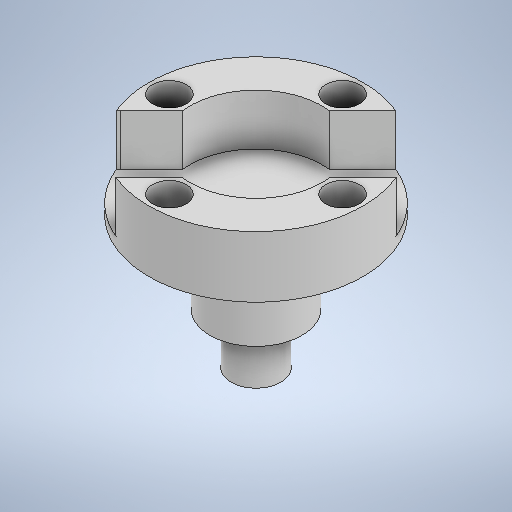
# Autodesk Inventor part: spinner
Saved by Autodesk Inventor 2025.1 (Build 291241000, 241)
## iProperties
Created: 2024-09-30
Part Number: spinner
Material: Generic
Document SubType Name: Modeling
Designer: m_kni
Density: 1 g/cm^3
Appearance: Default
Author: m_kni
Autodesk Inventor part; units mm, degrees
ref_plane "YZ Plane" through (0, 0, 0) normal (1, 0, 0) x (0, 1, 0)
ref_plane "XZ Plane" through (0, 0, 0) normal (0, 1, 0) x (-1, 0, 0)
ref_plane "XY Plane" through (0, 0, 0) normal (0, 0, 1) x (1, 0, 0)
sketch "Sketch1" plane through (0, 0, 0) normal (0, 1, 0) x (-1, 0, 0)
  line L0 (-12.7, 12.7) -> (12.7, 12.7)
  line L1 (12.7, 12.7) -> (12.7, -12.7)
  line L2 (12.7, -12.7) -> (-12.7, -12.7)
  line L3 (-12.7, -12.7) -> (-12.7, 12.7)
  line L4 (-12.7, 12.7) -> (12.7, -12.7) construction
  line L5 (12.7, 12.7) -> (-12.7, -12.7) construction
  line L6 (-11.4786, 11.4786) -> (11.4786, 11.4786)
  line L7 (11.4786, 11.4786) -> (11.4786, -11.4786)
  line L8 (11.4786, -11.4786) -> (-11.4786, -11.4786)
  line L9 (-11.4786, -11.4786) -> (-11.4786, 11.4786)
  line L10 (-11.4786, 11.4786) -> (11.4786, -11.4786) construction
  line L11 (11.4786, 11.4786) -> (-11.4786, -11.4786) construction
  line L12 (-25.4, -25.4) -> (25.4, -25.4)
  line L13 (25.4, -25.4) -> (25.4, 25.4)
  line L14 (25.4, 25.4) -> (-25.4, 25.4)
  line L15 (-25.4, 25.4) -> (-25.4, -25.4)
  line L16 (-25.4, -25.4) -> (25.4, 25.4) construction
  line L17 (25.4, -25.4) -> (-25.4, 25.4) construction
  circle A0 centre (0, 0) radius 5.5
  circle A1 centre (11.4786, 11.4786) radius 5.5
  circle A2 centre (11.4786, -11.4786) radius 5.5
  circle A3 centre (-11.4786, 11.4786) radius 5.5
  circle A4 centre (-11.4786, -11.4786) radius 5.5
  circle A5 centre (-25.4, 25.4) radius 5.5
  circle A6 centre (25.4, 25.4) radius 5.5
  circle A7 centre (25.4, -25.4) radius 5.5
  circle A8 centre (-25.4, -25.4) radius 5.5
  line L18 (7.5895, 15.3677) -> (21.5109, 29.2891)
  line L19 (29.2891, 21.5109) -> (15.3677, 7.5895)
  line L20 (15.3677, -7.5895) -> (29.2891, -21.5109)
  line L21 (-7.5895, -15.3677) -> (-21.5109, -29.2891)
  line L22 (-29.2891, 21.5109) -> (-15.3677, 7.5895)
  line L23 (7.5895, -15.3677) -> (21.5109, -29.2891)
  line L24 (-14.6585, -6.991) -> (-28.5798, -20.9124)
  line L25 (-8.9306, 16.3528) -> (-21.4569, 29.2343)
  line L26 (-35, -35) -> (35, -35)
  line L27 (35, -35) -> (35, 35)
  line L28 (35, 35) -> (-35, 35)
  line L29 (-35, 35) -> (-35, -35)
  line L30 (-35, -35) -> (35, 35) construction
  line L31 (35, -35) -> (-35, 35) construction
  circle A9 centre (11.4786, 11.4786) radius 2.5
  circle A10 centre (25.4, 25.4) radius 2.5
  line L32 (27.1678, 23.6322) -> (13.2464, 9.7109)
  line L33 (23.7072, 27.2397) -> (9.7111, 13.2466)
  line L34 (0, 0) -> (0, 35)
  line L35 (35, 0) -> (0, 0)
  line L36 (-27.1678, 23.6322) -> (-13.2464, 9.7109)
  circle A11 centre (-25.4, 25.4) radius 2.5
  line L37 (-23.7072, 27.2397) -> (-9.7111, 13.2466)
  circle A12 centre (-11.4786, 11.4786) radius 2.5
  circle A13 centre (25.4, -25.4) radius 2.5
  line L38 (23.7072, -27.2397) -> (9.7111, -13.2466)
  line L39 (27.1678, -23.6322) -> (13.2464, -9.7109)
  circle A14 centre (11.4786, -11.4786) radius 2.5
  circle A15 centre (-11.4786, -11.4786) radius 2.5
  line L40 (-23.7072, -27.2397) -> (-9.7111, -13.2466)
  line L41 (-27.1678, -23.6322) -> (-13.2464, -9.7109)
  line L42 (25.4, 25.4) -> (-25.4, -25.4) construction
  circle A16 centre (-25.4, -25.4) radius 2.5
  circle A17 centre (0, 0) radius 10.5
  circle A18 centre (0, 0) radius 6.5
  dimension "d0" = 25.4
  dimension "d1" = 25.4
  dimension "d2" = 50.8
  dimension "d3" = 50.8
  dimension "d4" = 11
  dimension "d5" = 11
  dimension "d6" = 11
  dimension "d7" = 11
  dimension "d8" = 11
  dimension "d9" = 11
  dimension "d10" = 11
  dimension "d11" = 11
  dimension "d12" = 11
  dimension "d13" = 70
  dimension "d14" = 5
  dimension "d15" = 5
  dimension "d16" = 21
  dimension "d17" = 13
  constraints: 86 end point, 32 point on circle, 19 centre point, 18 symmetric about line, 14 coincident, 13 tangent, 10 midpoint, 8 parallel, 5 horizontal, 5 perpendicular, 3 point on line, 6 other
  measures "d0" distance of L1.end L2.end
  measures "d1" distance of L0.end L1.end
  measures "d2" distance of L14.end L13.end
  measures "d3" distance of L13.end L12.end
  measures "d4" diameter of A0
  measures "d5" diameter of A1
  measures "d6" diameter of A2
  measures "d7" diameter of A3
  measures "d8" diameter of A4
  measures "d9" diameter of A5
  measures "d10" diameter of A6
  measures "d11" diameter of A7
  measures "d12" diameter of A8
  measures "d13" distance of L28.end L27.end
  measures "d14" diameter of A9
  measures "d15" diameter of A10
  measures "d16" diameter of A17
  measures "d17" diameter of A18
extrude "Extrusion1" add sketch "Sketch1" along normal blind 8 contours A18 L35 A0 L34 | L34 A0 L35 A18 | L34 L35 A0 | A0 L35 L34
sketch "Sketch2" plane through (0, 8, 0) normal (0, 1, 0) x (1, 0, 0)
  line L0 (-12.7, 12.7) -> (12.7, 12.7)
  line L1 (12.7, 12.7) -> (12.7, -12.7)
  line L2 (12.7, -12.7) -> (-12.7, -12.7)
  line L3 (-12.7, -12.7) -> (-12.7, 12.7)
  line L4 (-12.7, 12.7) -> (12.7, -12.7) construction
  line L5 (12.7, 12.7) -> (-12.7, -12.7) construction
  line L6 (-11.4786, 11.4786) -> (11.4786, 11.4786)
  line L7 (11.4786, 11.4786) -> (11.4786, -11.4786)
  line L8 (11.4786, -11.4786) -> (-11.4786, -11.4786)
  line L9 (-11.4786, -11.4786) -> (-11.4786, 11.4786)
  line L10 (-11.4786, 11.4786) -> (11.4786, -11.4786) construction
  line L11 (11.4786, 11.4786) -> (-11.4786, -11.4786) construction
  line L12 (-25.4, -25.4) -> (25.4, -25.4)
  line L13 (25.4, -25.4) -> (25.4, 25.4)
  line L14 (25.4, 25.4) -> (-25.4, 25.4)
  line L15 (-25.4, 25.4) -> (-25.4, -25.4)
  line L16 (-25.4, -25.4) -> (25.4, 25.4) construction
  line L17 (25.4, -25.4) -> (-25.4, 25.4) construction
  circle A0 centre (0, 0) radius 5.5
  circle A1 centre (11.4786, 11.4786) radius 5.5
  circle A2 centre (11.4786, -11.4786) radius 5.5
  circle A3 centre (-11.4786, 11.4786) radius 5.5
  circle A4 centre (-11.4786, -11.4786) radius 5.5
  circle A5 centre (-25.4, 25.4) radius 5.5
  circle A6 centre (25.4, 25.4) radius 5.5
  circle A7 centre (25.4, -25.4) radius 5.5
  circle A8 centre (-25.4, -25.4) radius 5.5
  line L18 (7.5895, 15.3677) -> (21.5109, 29.2891)
  line L19 (29.2891, 21.5109) -> (15.3677, 7.5895)
  line L20 (15.3677, -7.5895) -> (29.2891, -21.5109)
  line L21 (-7.5895, -15.3677) -> (-21.5109, -29.2891)
  line L22 (-29.2891, 21.5109) -> (-15.3677, 7.5895)
  line L23 (7.5895, -15.3677) -> (21.5109, -29.2891)
  line L24 (-16.1952, -8.6495) -> (-30.1166, -22.5709)
  line L25 (-9.6329, 16.6597) -> (-21.393, 29.1675)
  line L26 (-35, -35) -> (35, -35)
  line L27 (35, -35) -> (35, 35)
  line L28 (35, 35) -> (-35, 35)
  line L29 (-35, 35) -> (-35, -35)
  line L30 (-35, -35) -> (35, 35) construction
  line L31 (35, -35) -> (-35, 35) construction
  circle A9 centre (11.4786, 11.4786) radius 2.5
  circle A10 centre (25.4, 25.4) radius 2.5
  line L32 (27.1678, 23.6322) -> (13.2464, 9.7109)
  line L33 (23.5125, 27.0393) -> (9.7114, 13.247)
  line L34 (0, 0) -> (0, 35)
  line L35 (35, 0) -> (0, 0)
  line L36 (-27.1678, 23.6322) -> (-13.2464, 9.7109)
  circle A11 centre (-25.4, 25.4) radius 2.5
  line L37 (-23.5125, 27.0393) -> (-9.7114, 13.247)
  circle A12 centre (-11.4786, 11.4786) radius 2.5
  circle A13 centre (25.4, -25.4) radius 2.5
  line L38 (23.5125, -27.0393) -> (9.7114, -13.247)
  line L39 (27.1678, -23.6322) -> (13.2464, -9.7109)
  circle A14 centre (11.4786, -11.4786) radius 2.5
  circle A15 centre (-11.4786, -11.4786) radius 2.5
  line L40 (-23.5125, -27.0393) -> (-9.7114, -13.247)
  line L41 (-27.1678, -23.6322) -> (-13.2464, -9.7109)
  line L42 (25.4, 25.4) -> (-25.4, -25.4) construction
  circle A16 centre (-25.4, -25.4) radius 2.5
  circle A17 centre (0, 0) radius 10.5
  dimension "d20" = 25.4
  dimension "d21" = 25.4
  dimension "d22" = 50.8
  dimension "d23" = 50.8
  dimension "d24" = 11
  dimension "d25" = 11
  dimension "d26" = 11
  dimension "d27" = 11
  dimension "d28" = 11
  dimension "d29" = 11
  dimension "d30" = 11
  dimension "d31" = 11
  dimension "d32" = 11
  dimension "d33" = 70
  dimension "d34" = 5
  dimension "d35" = 5
  dimension "d36" = 21
  constraints: 86 end point, 32 point on circle, 18 centre point, 18 symmetric about line, 13 coincident, 13 tangent, 10 midpoint, 8 parallel, 5 horizontal, 5 perpendicular, 3 point on line, 6 other
  measures "d20" distance of L1.end L2.end
  measures "d21" distance of L0.end L1.end
  measures "d22" distance of L14.end L13.end
  measures "d23" distance of L13.end L12.end
  measures "d24" diameter of A0
  measures "d25" diameter of A1
  measures "d26" diameter of A2
  measures "d27" diameter of A3
  measures "d28" diameter of A4
  measures "d29" diameter of A5
  measures "d30" diameter of A6
  measures "d31" diameter of A7
  measures "d32" diameter of A8
  measures "d33" distance of L28.end L27.end
  measures "d34" diameter of A9
  measures "d35" diameter of A10
  measures "d36" diameter of A17
extrude "Extrusion2" add sketch "Sketch2" along normal blind 6 contours A17 L35 A0 L34 | L34 A0 L35 A17 | L34 L35 A0 | A0 L35 L34
sketch "Sketch3" plane through (0, 8, 0) normal (0, -1, 0) x (1, 0, 0)
  circle A0 centre (0, -8.5) radius 1.65
  circle A1 centre (8.5, 0) radius 1.65
  circle A2 centre (-8.5, 0) radius 1.65
  circle A3 centre (0, 8.5) radius 1.65
  point P0 (0, 0)
  dimension "d39" = 8.5
  dimension "d40" = 8.5
  dimension "d41" = 8.5
  dimension "d42" = 8.5
  dimension "d43" = 3.3
  dimension "d44" = 3.3
  dimension "d45" = 3.3
  dimension "d46" = 3.3
  constraints: 4 centre point, 4 coincident
  measures "d39" distance of point (0, -8.5) point (0, 0)
  measures "d40" distance of point (-8.5, 0) point (0, 0)
  measures "d41" distance of point (0, 8.5) point (0, 0)
  measures "d42" distance of point (8.5, 0) point (0, 0)
  measures "d43" diameter of A0
  measures "d44" diameter of A1
  measures "d45" diameter of A2
  measures "d46" diameter of A3
extrude "Extrusion3" cut sketch "Sketch3" against normal blind 6
sketch "Sketch4" plane through (0, 0, 0) normal (0, -1, 0) x (1, 0, 0)
  circle A0 centre (0, 0) radius 2.45
  dimension "d49" = 4.9
  constraints: 1 centre point, 1 coincident
  measures "d49" diameter of A0
extrude "Extrusion4" add sketch "Sketch4" along normal blind 5
sketch "Sketch5" plane through (0, 0, 0) normal (0, -1, 0) x (1, 0, 0)
  circle A0 centre (0, 0) radius 4.5
  circle A1 centre (0, 0) radius 6.5
  dimension "d52" = 9
  constraints: 2 centre point, 2 coincident
  measures "d52" diameter of A0
extrude "Extrusion5" cut sketch "Sketch5" against normal blind 12
sketch "Sketch8" plane through (0, 14, 0) normal (0, 1, 0) x (1, 0, 0)
  circle A0 centre (0, 0) radius 1.5
  circle A1 centre (0, 0) radius 5.6
  line L0 (-8.3358, -3.9626) -> (-17.8155, -2.4306)
  arc A2 (-17.8155, 2.5054) -> (-17.8155, -2.4306) centre (-17.4166, 0.0374) ccw
  line L1 (-8.3358, 4.0374) -> (-17.8155, 2.5054)
  line L2 (8.5026, 4.0374) -> (17.9822, 2.5054)
  arc A3 (17.9822, -2.4306) -> (17.9822, 2.5054) centre (17.5834, 0.0374) ccw
  line L3 (8.5026, -3.9626) -> (17.9822, -2.4306)
  line L4 (-8.3358, 4.0374) -> (-17.8155, 2.5054)
  line L5 (-17.8155, -2.4306) -> (-8.3358, -3.9626)
  line L6 (17.9822, 2.5054) -> (8.5026, 4.0374)
  line L7 (8.5026, -3.9626) -> (17.9822, -2.4306)
  circle A4 centre (17.5834, 0.0374) radius 2.5
  circle A5 centre (-17.4166, 0.0374) radius 2.5
  circle A6 centre (0, 0) radius 10.5
  line L8 (-3.0923, -8.6963) -> (-4.0736, -9.6776)
  line L9 (-8.7492, -3.0394) -> (-9.7087, -3.999)
  line L10 (8.8142, 3.2102) -> (9.6776, 4.0736)
  line L11 (3.1574, 8.8671) -> (3.999, 9.7087)
  line L12 (-4.0736, -9.6776) -> (0, -5.6)
  line L13 (-9.7087, -3.999) -> (-6.4572, -0.7443)
  circle A7 centre (0, 0) radius 6.5 projected
  line L14 (3.999, 9.7087) -> (-0.1204, 5.5987)
  line L15 (9.6776, 4.0736) -> (5.6, 0.0055)
  circle A8 centre (0, 0) radius 6.5
  point P0 (-0.8441, -6.445)
  point P1 (6.4444, 0.848)
  point P2 (0.7405, 6.4577)
  point P3 (-9.4866, -3.7766)
  point P4 (-9.4864, -3.7767)
  constraints: 32 end point, 11 point on circle, 8 centre point, 7 coincident, 5 point on line, 3 parallel, 2 concentric, 1 collinear, 3 other
extrude "Extrusion7" cut sketch "Sketch8" against normal blind 5 contours A0 | A1 | A1 L15 A7 L12 | A1 L14 A7 L15 | L12 A7 L14 A1 | A7 L14 L11 A6 L10 L15 | L12 L8 A6 L9 L13 A7
sketch "Sketch9" plane through (0, 9, 0) normal (0, 1, 0) x (1, 0, 0)
  circle A0 centre (0, 0) radius 6.5
  circle A1 centre (0, 0) radius 4.4883
  constraints: 2 centre point, 2 coincident
extrude "Extrusion8" add sketch "Sketch9" against normal up to surface (1 mm away)
sketch "Sketch10" plane through (0, -5, 0) normal (0, -1, 0) x (1, 0, 0)
  point P0 (0, 0)
body "Solid1"
